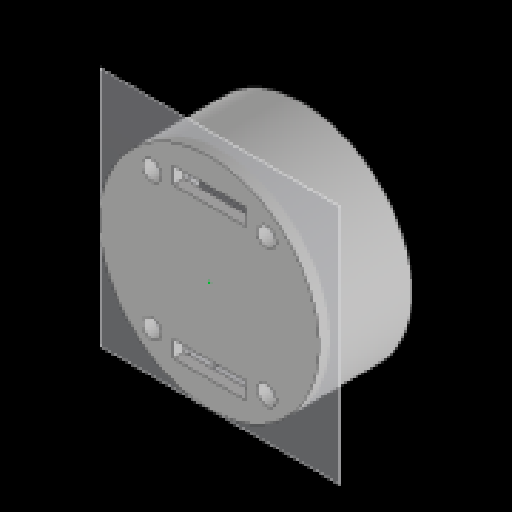
# Autodesk Inventor part: colorSensorHolder
Saved by Autodesk Inventor 2024.3 (Build 283343010, 343A)
## iProperties
Created: 2025-05-28
Part Number: colorSensorHolder
Material: Generic
Document SubType Name: Modeling
Designer: Oleg Kelner
Density: 1 g/cm^3
Appearance: Default
Author: Oleg Kelner
Autodesk Inventor part; units mm, degrees
ref_plane "YZ Plane" through (0, 0, 0) normal (1, 0, 0) x (0, 1, 0)
ref_plane "XZ Plane" through (0, 0, 0) normal (0, 1, 0) x (-1, 0, 0)
ref_plane "XY Plane" through (0, 0, 0) normal (0, 0, 1) x (1, 0, 0)
ref_plane "Work Plane2" through (0, 0, 0) normal (0, 0, 1) x (1, 0, 0)
sketch "Sketch2" plane through (0, 0, 0) normal (0, 0, 1) x (1, 0, 0)
  arc A0 (4.525, -18.0412) -> (4.525, 18.0412) centre (0, 0) ccw construction
  line L0 (4.525, 18.0412) -> (4.525, 18.3) construction
  line L1 (4.525, 18.3) -> (-4.525, 18.3) construction
  line L2 (-4.525, 18.3) -> (-4.525, 18.0412) construction
  arc A1 (-4.525, 18.0412) -> (-4.525, -18.0412) centre (0, 0) ccw construction
  line L3 (-4.525, -18.0412) -> (-4.525, -18.3) construction
  line L4 (-4.525, -18.3) -> (4.525, -18.3) construction
  line L5 (4.525, -18.3) -> (4.525, -18.0412) construction
  circle A2 centre (-10.45, -12.5) radius 1.5 construction
  circle A3 centre (-10.45, 12.5) radius 1.5 construction
  circle A4 centre (10.45, -12.5) radius 1.5 construction
  circle A5 centre (10.45, 12.5) radius 1.5 construction
  line L6 (-6.3484, -12.46) -> (6.3516, -12.46) construction
  line L7 (6.3516, -12.46) -> (6.3516, -15) construction
  line L8 (6.3516, -15) -> (-6.3484, -15) construction
  line L9 (-6.3484, -15) -> (-6.3484, -12.46) construction
  line L10 (6.3516, 15) -> (6.3516, 12.46) construction
  line L11 (6.3516, 12.46) -> (-6.3484, 12.46) construction
  line L12 (-6.3484, 12.46) -> (-6.3484, 15) construction
  line L13 (-6.3484, 15) -> (6.3516, 15) construction
  line L14 (6.6016, -12.21) -> (-6.5984, -12.21)
  line L15 (-6.5984, -12.21) -> (-6.5984, -15.25)
  line L16 (-6.5984, -15.25) -> (6.6016, -15.25)
  line L17 (6.6016, -15.25) -> (6.6016, -12.21)
  line L18 (-6.5984, 12.21) -> (6.6016, 12.21)
  line L19 (6.6016, 12.21) -> (6.6016, 15.25)
  line L20 (6.6016, 15.25) -> (-6.5984, 15.25)
  line L21 (-6.5984, 15.25) -> (-6.5984, 12.21)
  circle A6 centre (-10.45, -12.5) radius 1.75
  circle A7 centre (-10.45, 12.5) radius 1.75
  circle A8 centre (10.45, -12.5) radius 1.75
  circle A9 centre (10.45, 12.5) radius 1.75
  circle A10 centre (0, 0) radius 20
  point P0 (0, 0)
  dimension "d1" = 0.25
  dimension "d2" = 0.25
  dimension "d3" = 0.25
  dimension "d4" = 0.25
  dimension "d5" = 0.25
  dimension "d6" = 0.25
  dimension "d7" = 40
  constraints: 16 end point, 5 centre point, 1 coincident, 6 other
  measures "d1" distance between parallel lines of L6 L14
  measures "d2" distance between parallel lines of L11 L18
  measures "d3" radial gap between concentric circles of A2 A6
  measures "d4" radial gap between concentric circles of A3 A7
  measures "d5" radial gap between concentric circles of A4 A8
  measures "d6" radial gap between concentric circles of A5 A9
  measures "d7" diameter of A10
extrude "Extrusion1" add sketch "Sketch2" along normal blind 2
sketch "Sketch3" plane through (0, 0, 0) normal (0, 0, -1) x (-1, 0, 0)
  arc A0 (-4.525, 18.0412) -> (-4.525, -18.0412) centre (0, 0) ccw construction
  line L0 (-4.525, -18.0412) -> (-4.525, -18.3) construction
  line L1 (-4.525, -18.3) -> (4.525, -18.3) construction
  line L2 (4.525, -18.3) -> (4.525, -18.0412) construction
  arc A1 (4.525, -18.0412) -> (4.525, 18.0412) centre (0, 0) ccw construction
  line L3 (4.525, 18.0412) -> (4.525, 18.3) construction
  line L4 (4.525, 18.3) -> (-4.525, 18.3) construction
  line L5 (-4.525, 18.3) -> (-4.525, 18.0412) construction
  line L6 (5.3784, 13.43) -> (4.7784, 13.43) construction
  line L7 (4.7784, 13.43) -> (4.7784, 14.03) construction
  line L8 (4.7784, 14.03) -> (5.3784, 14.03) construction
  line L9 (5.3784, 14.03) -> (5.3784, 13.43) construction
  line L10 (0.2984, 13.43) -> (-0.3016, 13.43) construction
  line L11 (-0.3016, 13.43) -> (-0.3016, 14.03) construction
  line L12 (-0.3016, 14.03) -> (0.2984, 14.03) construction
  line L13 (0.2984, 14.03) -> (0.2984, 13.43) construction
  line L14 (-4.7816, 14.03) -> (-4.7816, 13.43) construction
  line L15 (-4.7816, 13.43) -> (-5.3816, 13.43) construction
  line L16 (-5.3816, 13.43) -> (-5.3816, 14.03) construction
  line L17 (-5.3816, 14.03) -> (-4.7816, 14.03) construction
  line L18 (-2.2416, 14.03) -> (-2.2416, 13.43) construction
  line L19 (-2.2416, 13.43) -> (-2.8416, 13.43) construction
  line L20 (-2.8416, 13.43) -> (-2.8416, 14.03) construction
  line L21 (-2.8416, 14.03) -> (-2.2416, 14.03) construction
  line L22 (2.8384, 13.43) -> (2.2384, 13.43) construction
  line L23 (2.2384, 13.43) -> (2.2384, 14.03) construction
  line L24 (2.2384, 14.03) -> (2.8384, 14.03) construction
  line L25 (2.8384, 14.03) -> (2.8384, 13.43) construction
  line L26 (4.7784, -13.43) -> (5.3784, -13.43) construction
  line L27 (5.3784, -13.43) -> (5.3784, -14.03) construction
  line L28 (5.3784, -14.03) -> (4.7784, -14.03) construction
  line L29 (4.7784, -14.03) -> (4.7784, -13.43) construction
  line L30 (-0.3016, -13.43) -> (0.2984, -13.43) construction
  line L31 (0.2984, -13.43) -> (0.2984, -14.03) construction
  line L32 (0.2984, -14.03) -> (-0.3016, -14.03) construction
  line L33 (-0.3016, -14.03) -> (-0.3016, -13.43) construction
  line L34 (-4.7816, -13.43) -> (-4.7816, -14.03) construction
  line L35 (-4.7816, -14.03) -> (-5.3816, -14.03) construction
  line L36 (-5.3816, -14.03) -> (-5.3816, -13.43) construction
  line L37 (-5.3816, -13.43) -> (-4.7816, -13.43) construction
  line L38 (-2.2416, -13.43) -> (-2.2416, -14.03) construction
  line L39 (-2.2416, -14.03) -> (-2.8416, -14.03) construction
  line L40 (-2.8416, -14.03) -> (-2.8416, -13.43) construction
  line L41 (-2.8416, -13.43) -> (-2.2416, -13.43) construction
  line L42 (2.2384, -13.43) -> (2.8384, -13.43) construction
  line L43 (2.8384, -13.43) -> (2.8384, -14.03) construction
  line L44 (2.8384, -14.03) -> (2.2384, -14.03) construction
  line L45 (2.2384, -14.03) -> (2.2384, -13.43) construction
  circle A2 centre (10.45, -12.5) radius 1.5 construction
  circle A3 centre (10.45, 12.5) radius 1.5 construction
  circle A4 centre (-10.45, -12.5) radius 1.5 construction
  circle A5 centre (-10.45, 12.5) radius 1.5 construction
  circle A6 centre (5.5, 6) radius 2.75 construction
  circle A7 centre (5.5, -6) radius 2.75 construction
  circle A8 centre (-5.5, 6) radius 2.75 construction
  circle A9 centre (-5.5, -6) radius 2.75 construction
  arc A10 (4.775, -18.2352) -> (4.775, 18.2352) centre (0, 0) ccw
  line L46 (4.775, -18.2352) -> (4.775, -18.55)
  line L47 (4.775, -18.55) -> (-4.775, -18.55)
  line L48 (-4.775, -18.55) -> (-4.775, -18.2352)
  arc A11 (-4.775, 18.2352) -> (-4.775, -18.2352) centre (0, 0) ccw
  line L49 (-4.775, 18.2352) -> (-4.775, 18.55)
  line L50 (-4.775, 18.55) -> (4.775, 18.55)
  line L51 (4.775, 18.55) -> (4.775, 18.2352)
  circle A12 centre (0, 0) radius 20 projected
  point P0 (0, 0)
  dimension "d10" = 0.25
  constraints: 12 end point, 4 point on circle, 2 centre point, 7 other
  measures "d10" radial gap between concentric circles of A1 A10
extrude "Extrusion2" add sketch "Sketch3" along normal blind 15
sketch "Sketch4" plane through (0, 0, 0) normal (0, 0, -1) x (-1, 0, 0)
  circle A0 centre (10.45, 12.5) radius 1.75 projected
  circle A1 centre (-10.45, 12.5) radius 1.75 projected
  circle A2 centre (10.45, -12.5) radius 1.75 projected
  circle A3 centre (-10.45, -12.5) radius 1.75 projected
  circle A4 centre (10.45, 12.5) radius 3.25
  circle A5 centre (10.45, -12.5) radius 3.25
  circle A6 centre (-10.45, -12.5) radius 3.25
  circle A7 centre (-10.45, 12.5) radius 3.25
  point P0 (0, 0)
  dimension "d13" = 1.5
  dimension "d14" = 1.5
  dimension "d15" = 1.5
  dimension "d16" = 1.5
  constraints: 4 centre point
  measures "d13" radial gap between concentric circles of A0 A4
  measures "d14" radial gap between concentric circles of A2 A5
  measures "d15" radial gap between concentric circles of A3 A6
  measures "d16" radial gap between concentric circles of A1 A7
extrude "Extrusion3" add sketch "Sketch4" along normal blind 2
fillet "Fillet1" radius 2 8 edges at (13.6635, 12.9858, -1) (10.3586, 15.7487, -1) (-10.3586, 15.7487, -1) (-13.6635, 12.9858, -1) (-13.6635, -12.9858, -1) (-10.3586, -15.7487, -1) (10.3586, -15.7487, -1) (13.6635, -12.9858, -1)
sketch "Sketch7" plane through (0, 0, 0) normal (0, 0, -1) x (-1, 0, 0)
  circle A0 centre (-12.5, 3.75) radius 1.6 construction
  circle A1 centre (-12.5, -3.75) radius 1.6 construction
  point P0 (0, 0)
hole "Hole1" at (12.5, -3.75, 0) at (12.5, 3.75, 0) direction (0, 0, 1) diameter 3.2 end through all countersink diameter 6 countersink angle 90
body "Solid1"
